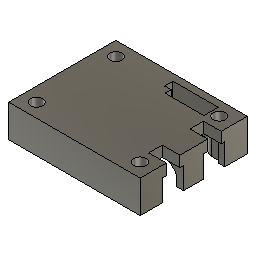
cover switch module (Autodesk Fusion 360 design; units mm, degrees)
Autodesk Fusion 360 part; units mm, degrees
note: some values were not read from the file. Set by a fixed rule: which sketch regions a step uses.
sketch "Skizze1" plane through (0, 0, 0) normal (0, 0, 1) x (1, 0, 0)
  line L0 (24.25, -19.75) -> (-24.25, -19.75)
  line L1 (-24.25, -19.75) -> (-24.25, 19.75)
  line L2 (-24.25, 19.75) -> (24.25, 19.75)
  line L3 (24.25, 19.75) -> (24.25, -19.75)
  line L4 (24.25, -19.75) -> (-24.25, 19.75) construction
  line L5 (-24.25, -19.75) -> (24.25, 19.75) construction
  dimension "d1" = 48.5
  dimension "d2" = 39.5
  constraint horizontal L0
  constraint perpendicular L0 L1
  constraint parallel L0 L2
  constraint parallel L1 L3
  constraint coincident L4 origin
  constraint coincident L5 origin
  measures "d1" distance of L1.end L2.end
  measures "d2" distance of L0.end L1.end
extrude "Extrusion1" add sketch "Skizze1" along normal blind 12
sketch "Skizze2" plane through (0, 0, 0) normal (0, 0, -1) x (1, 0, 0)
  line L0 (-24.25, -19.75) -> (24.25, -19.75)
  line L1 (24.25, -19.75) -> (24.25, 19.75)
  line L2 (24.25, 19.75) -> (-24.25, 19.75)
  line L3 (-24.25, 19.75) -> (-24.25, -19.75)
  line L4 (-21.75, 17.25) -> (21.75, 17.25)
  line L5 (21.75, 17.25) -> (21.75, -17.25)
  line L6 (21.75, -17.25) -> (-21.75, -17.25)
  line L7 (-21.75, -17.25) -> (-21.75, 17.25)
  line L8 (-21.75, 17.25) -> (21.75, -17.25) construction
  line L9 (21.75, 17.25) -> (-21.75, -17.25) construction
  dimension "d5" = 43.5
  dimension "d6" = 34.5
  constraint horizontal L4
  constraint perpendicular L4 L5
  constraint parallel L4 L6
  constraint parallel L5 L7
  constraint coincident L8 origin
  constraint coincident L9 origin
  measures "d5" distance of L5.end L6.end
  measures "d6" distance of L4.end L5.end
extrude "Extrusion2" cut sketch "Skizze2" against normal up to surface (10.5 mm away) contours L4 L5 L6 L7
sketch "Skizze4" plane through (0, 0, 10.5) normal (0, 0, -1) x (1, 0, 0)
  line L0 (21.75, -17.25) -> (21.75, 17.25)
  line L1 (21.75, 17.25) -> (-21.75, 17.25)
  line L2 (-21.75, 17.25) -> (-21.75, -17.25)
  line L3 (-21.75, -17.25) -> (21.75, -17.25)
  line L4 (-21.75, -17.25) -> (-16.05, -17.25)
  line L5 (-16.05, -17.25) -> (-16.05, -14.605)
  line L6 (-19.05, -11.605) -> (-21.75, -11.605)
  line L7 (-21.75, -11.605) -> (-21.75, -17.25)
  line L8 (-21.75, 17.25) -> (-16.05, 17.25)
  line L9 (-16.05, 17.25) -> (-16.05, 14.605)
  line L10 (-19.05, 11.605) -> (-21.75, 11.605)
  line L11 (-21.75, 11.605) -> (-21.75, 17.25)
  line L12 (21.75, 17.25) -> (16.05, 17.25)
  line L13 (16.05, 17.25) -> (16.05, 14.605)
  line L14 (19.05, 11.605) -> (21.75, 11.605)
  line L15 (21.75, 11.605) -> (21.75, 17.25)
  line L16 (21.75, -17.25) -> (16.05, -17.25)
  line L17 (16.05, -17.25) -> (16.05, -14.605)
  line L18 (19.05, -11.605) -> (21.75, -11.605)
  line L19 (21.75, -11.605) -> (21.75, -17.25)
  arc A0 (-19.05, 11.605) -> (-16.05, 14.605) centre (-19.05, 14.605) ccw
  arc A1 (16.05, 14.605) -> (19.05, 11.605) centre (19.05, 14.605) ccw
  arc A2 (19.05, -11.605) -> (16.05, -14.605) centre (19.05, -14.605) ccw
  arc A3 (-16.05, -14.605) -> (-19.05, -11.605) centre (-19.05, -14.605) ccw
  dimension "d9" = 3
  dimension "d10" = 29.21
  dimension "d11" = 38.1
  constraint horizontal L4
  constraint vertical L5
  constraint horizontal L6
  constraint vertical L7
  constraint coincident L2.end L3.start
  constraint horizontal L8
  constraint vertical L9
  constraint horizontal L10
  constraint vertical L11
  constraint coincident L1.end L2.start
  constraint horizontal L12
  constraint vertical L13
  constraint horizontal L14
  constraint vertical L15
  constraint coincident L0.end L1.start
  constraint horizontal L16
  constraint vertical L17
  constraint horizontal L18
  constraint vertical L19
  constraint coincident L0.start L3.end
  constraint tangent L9 A0
  constraint tangent L10 A0
  constraint tangent L13 A1
  constraint tangent L14 A1
  constraint equal A0 A1
  constraint tangent L17 A2
  constraint tangent L18 A2
  constraint equal A0 A2
  constraint tangent L5 A3
  constraint tangent L6 A3
  constraint equal A0 A3
  constraint collinear L6 L18
  constraint collinear L10 L14
  constraint collinear L5 L9
  constraint collinear L13 L17
  constraint equal L10 L14
  constraint equal L5 L9
  measures "d9" radius of A0
  measures "d10" distance of A0.centre A3.centre
  measures "d11" distance of A2.centre A3.centre
extrude "Extrusion3" add sketch "Skizze4" along normal up to surface (9.75 mm away) contours L0 L3 L16 L17 L18 L19 A2 | L0 L1 L12 L13 L14 L15 A1 | L2 L3 L4 L5 L6 L7 A3 | L1 L2 L8 L9 L10 L11 A0
hole "Bohrung1" at (-19.05, -14.605, 12) direction (0, 0, -1) diameter 2.5 end through all counterbore diameter 4.5 counterbore depth 6
mirror "Spiegeln1" about plane through (0, 0, 0) normal (1, 0, 0) of "Bohrung1"
mirror "Spiegeln2" about plane through (0, 0, 0) normal (0, 1, 0) of "Bohrung1", "Spiegeln1"
sketch "Skizze5" plane through (24.25, 0, 0) normal (1, 0, 0) x (0, 1, 0)
  line L0 (-19.75, 12) -> (-19.75, 0)
  line L1 (-19.75, 0) -> (19.75, 0)
  line L2 (19.75, 0) -> (19.75, 12)
  line L3 (-3.77, 0) -> (-11.47, 0)
  line L4 (-11.47, 0) -> (-11.47, 8)
  line L5 (-11.47, 8) -> (-3.77, 8)
  line L6 (-3.77, 8) -> (-3.77, 0)
  line L7 (19.75, 12) -> (-19.75, 12)
  point P0 (-7.62, 0)
  dimension "d22" = 7.7
  dimension "d23" = 7.62
  dimension "d24" = 8
  constraint horizontal L3
  constraint vertical L4
  constraint horizontal L5
  constraint vertical L6
  constraint coincident L1 L3.start
  constraint midpoint L3 P0
  measures "d22" distance of L3.start L3.end
  measures "d23" distance of origin P0
  measures "d24" distance of L3.end L4.end
extrude "Extrusion4" cut sketch "Skizze5" against normal up to surface (2.5 mm away) contours L1 L3 L4 L5 L6
sketch "Skizze7" plane through (0, 0, 10.5) normal (0, 0, -1) x (1, 0, 0)
  line L0 (21.75, 11.605) -> (19.05, 11.605)
  arc A0 (16.05, 14.605) -> (19.05, 11.605) centre (19.05, 14.605) ccw
  line L1 (16.05, 14.605) -> (16.05, 17.25)
  line L2 (16.05, 17.25) -> (-16.05, 17.25)
  line L3 (-16.05, 17.25) -> (-16.05, 14.605)
  arc A1 (-19.05, 11.605) -> (-16.05, 14.605) centre (-19.05, 14.605) ccw
  line L4 (-19.05, 11.605) -> (-21.75, 11.605)
  line L5 (-21.75, 11.605) -> (-21.75, -11.605)
  line L6 (-21.75, -11.605) -> (-19.05, -11.605)
  arc A2 (-16.05, -14.605) -> (-19.05, -11.605) centre (-19.05, -14.605) ccw
  line L7 (-16.05, -14.605) -> (-16.05, -17.25)
  line L8 (-16.05, -17.25) -> (16.05, -17.25)
  line L9 (16.05, -17.25) -> (16.05, -14.605)
  arc A3 (19.05, -11.605) -> (16.05, -14.605) centre (19.05, -14.605) ccw
  line L10 (19.05, -11.605) -> (21.75, -11.605)
  line L11 (21.75, -11.605) -> (21.75, 11.605)
  line L12 (16.05, 14.605) -> (16.05, -14.605)
  constraint vertical L12
  constraint collinear L1 L12
  constraint coincident A0.start L1.start
  constraint coincident L9.end A3.end
extrude "Extrusion6" add sketch "Skizze7" along normal up to surface (2.5 mm away) contours L0 A0 A3 L10 L11 L12
sketch "Skizze6" plane through (24.25, 0, 0) normal (1, 0, 0) x (0, 1, 0)
  line L0 (-11.47, 0) -> (-11.47, 8)
  line L1 (-11.47, 8) -> (-3.77, 8)
  line L2 (-3.77, 8) -> (-3.77, 0)
  line L3 (-3.77, 0) -> (19.75, 0)
  line L4 (19.75, 0) -> (19.75, 12)
  line L5 (-19.75, 12) -> (-19.75, 0)
  line L6 (-19.75, 0) -> (-11.47, 0)
  line L7 (-10.12, 8) -> (-5.12, 8)
  line L8 (-5.12, 8) -> (-5.12, 12)
  line L9 (-5.12, 12) -> (-10.12, 12)
  line L10 (-10.12, 12) -> (-10.12, 8)
  line L11 (19.75, 12) -> (-19.75, 12)
  dimension "d27" = 5
  constraint horizontal L7
  constraint vertical L8
  constraint horizontal L9
  constraint vertical L10
  constraint coincident L1 L7.start
  constraint midpoint L1 L7
  constraint collinear L9 L11
  measures "d27" distance of L8.end L9.end
extrude "Extrusion5" cut sketch "Skizze6" against normal blind 6.5 contours L1 L7 L8 L9 L10 L11
mirror "Spiegeln5" about plane through (0, 0, 0) normal (0, 1, 0) of "Extrusion4", "Extrusion5"
sketch "Skizze8" plane through (-24.25, 0, 0) normal (-1, 0, 0) x (0, -1, 0)
  line L0 (-19.75, 12) -> (-19.75, 0)
  line L1 (-19.75, 0) -> (19.75, 0)
  line L2 (19.75, 0) -> (19.75, 12)
  line L3 (-11.5, 0) -> (11.5, 0)
  line L4 (11.5, 0) -> (11.5, 7)
  line L5 (11.5, 7) -> (-11.5, 7)
  line L6 (-11.5, 7) -> (-11.5, 0)
  line L7 (19.75, 12) -> (-19.75, 12)
  dimension "d35" = 23
  dimension "d36" = 7
  constraint horizontal L3
  constraint vertical L4
  constraint horizontal L5
  constraint vertical L6
  constraint coincident L1 L3.start
  constraint midpoint L1 L3
  measures "d35" distance of L4.end L5.end
  measures "d36" distance of L3.start L5.end
extrude "Extrusion7" cut sketch "Skizze8" against normal up to surface (2.5 mm away) contours L1 L3 L4 L5 L6
chamfer "Fase2" distance 4 angle 45 1 edges at (21.75, 0, 8)
fillet "Abrundung1" radius 3 2 edges at (21.75, 0, 4) (17.75, 0, 8)
sketch "Skizze15" plane through (0, 0, 10.5) normal (0, 0, -1) x (1, 0, 0)
  line L0 (16.05, -17.25) -> (16.05, 17.25)
  line L1 (16.05, 17.25) -> (-16.05, 17.25)
  line L2 (-16.05, 17.25) -> (-16.05, 14.605)
  arc A0 (-19.05, 11.605) -> (-16.05, 14.605) centre (-19.05, 14.605) ccw
  line L3 (-19.05, 11.605) -> (-21.75, 11.605)
  line L4 (-21.75, 11.605) -> (-21.75, -11.605)
  line L5 (-21.75, -11.605) -> (-19.05, -11.605)
  arc A1 (-16.05, -14.605) -> (-19.05, -11.605) centre (-19.05, -14.605) ccw
  line L6 (-16.05, -14.605) -> (-16.05, -17.25)
  line L7 (-16.05, -17.25) -> (16.05, -17.25)
  circle A2 centre (19.05, -14.605) radius 1.25
  line L8 (16.05, -11.96) -> (1.73, -11.96)
  line L9 (1.73, -11.96) -> (1.73, -17.25)
  line L10 (1.73, -17.25) -> (16.05, -17.25)
  line L11 (16.05, -17.25) -> (16.05, -11.96)
  line L12 (16.05, -11.96) -> (1.73, -17.25) construction
  line L13 (1.73, -11.96) -> (16.05, -17.25) construction
  line L14 (8.89, -14.605) -> (13.97, -14.605) construction
  line L15 (13.97, -14.605) -> (19.05, -14.605) construction
  line L16 (1.73, -14.205) -> (-0.67, -14.205)
  line L17 (-0.67, -14.205) -> (-0.67, -17.25)
  line L18 (-0.67, -17.25) -> (1.73, -17.25)
  line L19 (1.73, -17.25) -> (1.73, -14.205)
  point P0 (8.89, -14.605)
  point P1 (1.73, -14.605)
  dimension "d53" = 5.08
  dimension "d54" = 5.08
  dimension "d55" = 0.4
  dimension "d56" = 2.4
  constraint horizontal L8
  constraint perpendicular L8 L9
  constraint parallel L8 L10
  constraint parallel L9 L11
  constraint coincident L12 P0
  constraint coincident L13 P0
  constraint coincident L0.start L7.end
  constraint coincident P0 L14.start
  constraint horizontal L14
  constraint coincident A2.centre L15.end
  constraint horizontal L15
  constraint horizontal L16
  constraint vertical L17
  constraint horizontal L18
  constraint vertical L19
  constraint coincident L7 L17.end
  constraint coincident L9 L16.start
  constraint midpoint L9 P1
  measures "d53" distance of P0 L14.end
  measures "d54" distance of L14.end A2.centre
  measures "d55" distance of L16 P1
  measures "d56" distance of L16.start L16.end
extrude "Extrusion10" cut sketch "Skizze15" against normal through all contours L0 L7 L8 L9 L10 L11 L19 | L7 L9 L16 L17 L18 L19
sketch "Skizze16" plane through (0, 0, 10.5) normal (0, 0, -1) x (1, 0, 0)
  line L0 (1.73, -11.96) -> (16.05, -11.96)
  line L1 (16.05, -11.96) -> (16.05, 17.25)
  line L2 (16.05, 17.25) -> (-16.05, 17.25)
  line L3 (-16.05, 17.25) -> (-16.05, 14.605)
  arc A0 (-19.05, 11.605) -> (-16.05, 14.605) centre (-19.05, 14.605) ccw
  line L4 (-19.05, 11.605) -> (-21.75, 11.605)
  line L5 (-21.75, 11.605) -> (-21.75, -11.605)
  line L6 (-21.75, -11.605) -> (-19.05, -11.605)
  arc A1 (-16.05, -14.605) -> (-19.05, -11.605) centre (-19.05, -14.605) ccw
  line L7 (-16.05, -14.605) -> (-16.05, -17.25)
  line L8 (-16.05, -17.25) -> (-0.67, -17.25)
  line L9 (-0.67, -17.25) -> (-0.67, -14.205)
  line L10 (-0.67, -14.205) -> (1.73, -14.205)
  line L11 (1.73, -14.205) -> (1.73, -11.96)
  line L12 (14.05, -11.96) -> (14.05, -9.96)
  line L13 (14.05, -9.96) -> (-2.67, -9.96)
  line L14 (-2.67, -9.96) -> (-2.67, -17.25)
  dimension "d58" = 2
  dimension "d59" = 2
  dimension "d60" = 2
  constraint coincident L0 L12.start
  constraint perpendicular L0 L12
  constraint perpendicular L12 L13
  constraint coincident L8 L14.end
  constraint perpendicular L8 L14
  measures "d58" distance of L9 L14
  measures "d59" distance of L12.start L12.end
  measures "d60" distance of L1 L12
extrude "Extrusion11" add sketch "Skizze16" along normal blind 6 contours L0 L8 L9 L10 L11 L12 L13 L14
equation "d23 = ( 15.24 / 2 ) * 1 mm"
equation "d59 = d58"
